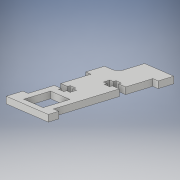
# Autodesk Inventor part: 板子10
Saved by Autodesk Inventor 2017 (Build 210142000, 142)
## iProperties
Part Number: 板子10
Material: 一般
Document SubType Name: Modeling
Designer: User
Density: 1 g/cm^3
Appearance: 預設
Author: User
Autodesk Inventor part; units mm, degrees
ref_plane "YZ Plane" through (0, 0, 0) normal (1, 0, 0) x (0, 1, 0)
ref_plane "XZ Plane" through (0, 0, 0) normal (0, 1, 0) x (-1, 0, 0)
ref_plane "XY Plane" through (0, 0, 0) normal (0, 0, 1) x (1, 0, 0)
sketch "草圖1" plane through (0, 0, 0) normal (0, 1, 0) x (-1, 0, 0)
  line L0 (5.5, -3) -> (-5.5, -3)
  line L1 (-5.5, -3) -> (-5.5, -15.75)
  line L2 (-5.5, -15.75) -> (5.5, -15.75)
  line L3 (5.5, -15.75) -> (5.5, -3)
  line L4 (-9, -39.5104) -> (-5, -39.5058)
  line L5 (-5, -39.5058) -> (-4.9985, -40.8058)
  line L6 (-4.9985, -40.8058) -> (-1.9985, -40.8023)
  line L7 (-1.9985, -40.8023) -> (-2, -39.5023)
  line L8 (-2, -39.5023) -> (0, -39.5)
  line L9 (-5, -35.2) -> (-2, -35.2)
  line L10 (-5, -36.5) -> (-5, -35.2)
  line L11 (-2, -35.2) -> (-2, -36.5)
  line L12 (-2, -36.5) -> (0, -36.5)
  line L13 (-9, -36.5) -> (-5, -36.5)
  line L14 (-12, 0) -> (-12, -5)
  line L15 (-12, -5) -> (-9, -5)
  line L16 (-9, -5) -> (-9, -36.5)
  line L17 (-12, 0) -> (-12, -5)
  line L18 (11.9851, -47) -> (8.9851, -47)
  line L19 (7.5982, -47) -> (9.4378, -47)
  arc A0 (7.5982, -47) -> (4.5816, -50.0166) centre (7.5982, -50.0166) ccw
  line L20 (0, -36.5) -> (0, -39.5)
  line L21 (-12, 0) -> (-12, -5)
  line L22 (-12, -5) -> (-9, -5)
  line L23 (-9, -5) -> (-9, -36.5)
  line L24 (-9, -36.5) -> (-5, -36.5)
  line L25 (-5, -36.5) -> (-5, -35.2)
  line L26 (-5, -35.2) -> (-2.2106, -35.2)
  line L27 (-5, -35.2) -> (-2, -35.2)
  line L28 (-2, -35.2) -> (-2, -36.5)
  line L29 (-2, -36.5) -> (0, -36.5)
  line L30 (0, -36.5) -> (0, -39.5)
  line L31 (0, -39.5) -> (-2, -39.5023)
  line L32 (-2, -39.5023) -> (-1.9985, -40.8023)
  line L33 (-1.9985, -40.8023) -> (-4.9985, -40.8058)
  line L34 (-4.9985, -40.8023) -> (-5, -39.5058)
  line L35 (-5, -39.5058) -> (-9, -39.5104)
  line L36 (-9, -39.5104) -> (-9, -52.5104)
  line L37 (-9, -52.5104) -> (-12.0184, -52.5104)
  line L38 (11.9851, -47) -> (7.5982, -47)
  line L39 (11.985, -7.9789) -> (11.985, 0)
  line L40 (11.985, 0) -> (-12, 0)
  line L41 (11.985, -7.9789) -> (8.985, -7.9789)
  line L42 (8.985, -7.9789) -> (8.985, -20.4789)
  line L43 (8.9851, -38) -> (11.9851, -38)
  line L44 (8.985, -20.4789) -> (4.985, -20.4789)
  line L45 (4.985, -20.4789) -> (4.985, -19.1789)
  line L46 (4.985, -19.1789) -> (1.985, -19.1789)
  line L47 (1.985, -19.1789) -> (1.985, -20.4789)
  line L48 (1.985, -20.4789) -> (-0.015, -20.4789)
  line L49 (-0.015, -20.4789) -> (-0.015, -23.4789)
  line L50 (1.985, -23.4789) -> (-0.015, -23.4789)
  line L51 (1.985, -23.4789) -> (1.985, -24.7789)
  line L52 (4.985, -24.7789) -> (1.985, -24.7789)
  line L53 (4.985, -24.7789) -> (4.985, -23.4789)
  line L54 (4.985, -23.5) -> (8.9851, -23.5)
  line L55 (8.9851, -23.5) -> (8.9851, -38)
  line L56 (11.9851, -38) -> (11.9851, -47)
  line L57 (4.5816, -50.0166) -> (4.5816, -60)
  line L58 (4.5816, -60) -> (-12.0184, -60)
  line L59 (-12.0184, -52.5104) -> (-12.0184, -60)
  point P0 (0, 0)
  dimension "d2" = 11
  dimension "d3" = 12.75
  dimension "d7" = 3
  dimension "d10" = 4
  dimension "d12" = 3
  dimension "d17" = 4
  dimension "d18" = 1.3
  dimension "d19" = 3
  dimension "d20" = 1.3
  dimension "d21" = 2
  dimension "d22" = 5
  dimension "d23" = 3
  dimension "d25" = 31.5
  dimension "d26" = 13
  dimension "d27" = 14.5
  dimension "d29" = 16.6
  dimension "d30" = 2
  constraints: 120 end point, 14 perpendicular, 10 horizontal, 9 vertical, 8 point on line, 7 collinear, 2 parallel, 2 point on circle, 1 centre point, 1 tangent
  measures "d2" distance of L0.start L0.end
  measures "d3" distance of L2.end L0.start
  measures "d7" distance of L39.start L41.end
  measures "d10" distance of L42.end L44.end
  measures "d12" distance of L45.end L46.end
  measures "d17" distance of L4.start L5.start
  measures "d18" distance of L5.start L6.start
  measures "d19" distance of L6.start L7.start
  measures "d20" distance of L7.start L8.start
  measures "d21" distance of L8.start L8.end
  measures "d22" distance of L14.start L14.end
  measures "d23" distance of L14.end L15.end
  measures "d25" distance from line of L15 L13.start
  measures "d26" distance of L4.start L36.end
  measures "d27" distance of L54.end L43.start
  measures "d29" distance of L57.end L58.end
  measures "d30" distance of L47.end L48.end
extrude "擠出1" add sketch "草圖1" along normal mid plane 3
